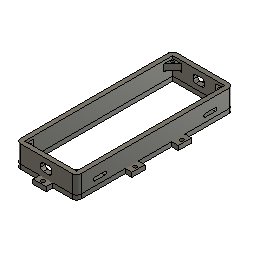
Electronics_Enclosure (Autodesk Fusion 360 design; units mm, degrees)
Autodesk Fusion 360 part; units mm, degrees
sketch "Sketch1" plane through (0, 0, 0) normal (0, 1, 0) x (1, 0, 0)
  line L0 (0, 0) -> (59.69, 0)
  line L1 (59.69, 0) -> (59.69, -170.18)
  line L2 (59.69, -170.18) -> (0, -170.18)
  line L3 (0, -170.18) -> (0, 0)
  line L4 (64.77, 5.08) -> (-5.08, 5.08)
  line L5 (-5.08, 5.08) -> (-5.08, -175.26)
  line L6 (-5.08, -175.26) -> (64.77, -175.26)
  line L7 (64.77, -175.26) -> (64.77, 5.08)
  line L8 (-5.08, -66.04) -> (-5.08, -50.8)
  line L9 (64.77, -85.09) -> (-5.08, -85.09) construction
  line L10 (-5.08, -66.04) -> (-5.08, -50.8)
  line L11 (29.845, -175.26) -> (29.845, 5.08) construction
  line L12 (64.77, -50.8) -> (72.39, -50.8)
  circle A0 centre (68.58, -58.42) radius 2.032
  line L13 (72.39, -50.8) -> (72.39, -66.04)
  line L14 (72.39, -66.04) -> (64.77, -66.04)
  line L15 (64.77, -119.38) -> (72.39, -119.38)
  line L16 (72.39, -119.38) -> (72.39, -104.14)
  line L17 (72.39, -104.14) -> (64.77, -104.14)
  circle A1 centre (68.58, -111.76) radius 2.032
  line L18 (37.465, 5.08) -> (22.225, 5.08)
  line L19 (22.225, 5.08) -> (22.225, 12.7)
  line L20 (22.225, 12.7) -> (37.465, 12.7)
  line L21 (37.465, 12.7) -> (37.465, 5.08)
  line L22 (29.845, 5.08) -> (29.845, 12.7) construction
  circle A2 centre (29.845, 8.89) radius 2.032
  line L23 (22.225, -175.26) -> (22.225, -182.88)
  line L24 (22.225, -182.88) -> (37.465, -182.88)
  line L25 (37.465, -182.88) -> (37.465, -175.26)
  circle A3 centre (29.845, -179.07) radius 2.032
  dimension "d1" = 170.18
  dimension "d2" = 59.69
  dimension "d3" = 5.08
  dimension "d4" = 5.08
  dimension "d5" = 5.08
  dimension "d6" = 5.08
  dimension "d11" = 15.24
  dimension "d12" = 7.62
  dimension "d13" = 4.064
  dimension "d44" = 15.24
  dimension "d45" = 7.62
  dimension "d46" = 7.62
  dimension "d47" = 15.24
  dimension "d48" = 38.1
  dimension "d49" = 55.88
  dimension "d50" = 7.62
  dimension "d51" = 3.81
  dimension "d52" = 4.064
  dimension "d53" = 4.064
  dimension "d54" = 7.62
  dimension "d55" = 3.81
  constraint horizontal L0
  constraint vertical L1
  constraint horizontal L2
  constraint vertical L3
  constraint coincident L0.start L3.end
  constraint horizontal L4
  constraint vertical L5
  constraint horizontal L6
  constraint vertical L7
  constraint vertical L8
  constraint coincident L5 L8.end
  constraint midpoint L7 L9.start
  constraint midpoint L5 L9.end
  constraint midpoint L6 L11.start
  constraint midpoint L4 L11.end
  constraint symmetric L8.end L11 L12.start
  constraint symmetric L8.start L11 L14.end
  constraint horizontal L18
  constraint vertical L19
  constraint horizontal L20
  constraint vertical L21
  constraint coincident L4 L18.start
  constraint midpoint L18 L11.end
  constraint midpoint L20 L22.end
  constraint coincident L11.end L22.start
  constraint midpoint L22 A2.centre
  constraint symmetric L9 L18.start L25.end
  constraint symmetric L9 L18.end L23.start
  constraint symmetric L9 L19.end L23.end
  constraint symmetric L9 L20.end L24.end
  constraint symmetric L9 A2 A3
  constraint perpendicular L7 L14
  constraint perpendicular L13 L14
  constraint perpendicular L7 L15
  constraint perpendicular L15 L16
  constraint coincident L7 L17.end
  measures "d1" distance of L0.start L2.end
  measures "d2" distance of L0.start L0.end
  measures "d3" distance of L1 L7
  measures "d4" distance of L3 L5
  measures "d5" distance of L2 L6
  measures "d6" distance of L0 L4
  measures "d11" distance of L18.start L18.end
  measures "d12" distance of L18.start L20.end
  measures "d13" diameter of A2
  measures "d44" distance of L12.end L13.end
  measures "d45" distance of L12.start L12.end
  measures "d46" distance of L16.end L17.end
  measures "d47" distance of L15.end L16.end
  measures "d48" distance of L14 L17
  measures "d49" distance of L4 L12
  measures "d50" distance of L15 A1.centre
  measures "d51" distance of L16 A1.centre
  measures "d52" diameter of A1
  measures "d53" diameter of A0
  measures "d54" distance of A0.centre L14
  measures "d55" distance of A0.centre L13
extrude "Extrude2" add sketch "Sketch1" along normal blind 5.08 makes body 1
extrude "Extrude1" add sketch "Sketch1" along normal blind 25.4 separate body contours L4 L5 L6 L7 L8 L10 L18 makes body 2
sketch "Sketch2" plane through (0, 25.4, 0) normal (0, 1, 0) x (-1, 0, 0)
  line L0 (-59.69, 170.18) -> (0, 170.18)
  line L1 (0, 170.18) -> (0, 0)
  line L2 (0, 0) -> (-59.69, 0)
  line L3 (-59.69, 0) -> (-59.69, 170.18)
  line L4 (5.08, -5.08) -> (5.08, 175.26)
  line L5 (5.08, 175.26) -> (-64.77, 175.26)
  line L6 (-64.77, 175.26) -> (-64.77, -5.08)
  line L7 (-64.77, -5.08) -> (5.08, -5.08)
ref_plane "WorkPlane1" through (29.845, 22.225, 85.09) normal (0, 1, 0) x (-1, 0, 0)
sketch "Sketch4" plane through (29.845, 22.225, 85.09) normal (0, 1, 0) x (1, 0, 0)
  line L0 (-29.845, 85.09) -> (29.845, 85.09)
  line L1 (29.845, 85.09) -> (29.845, -85.09)
  line L2 (19.685, 85.09) -> (29.845, 74.93)
  line L3 (29.845, 85.09) -> (19.685, 85.09)
  line L4 (29.845, -85.09) -> (19.685, -85.09)
  line L5 (19.685, -85.09) -> (29.845, -74.93)
  line L6 (29.845, -85.09) -> (29.845, -74.93)
  line L7 (-29.845, -85.09) -> (-29.845, 85.09)
  line L8 (-29.845, 85.09) -> (-19.685, 85.09)
  line L9 (-29.845, 85.09) -> (-29.845, 74.93)
  line L10 (-29.845, 74.93) -> (-19.685, 85.09)
  line L11 (29.845, -85.09) -> (-29.845, -85.09)
  line L12 (-29.845, -85.09) -> (-29.845, -74.93)
  line L13 (-29.845, -85.09) -> (-19.685, -85.09)
  line L14 (-19.685, -85.09) -> (-29.845, -74.93)
  circle A0 centre (26.9059, 82.1509) radius 1.651
  line L15 (29.845, 85.09) -> (24.765, 80.01) construction
  line L16 (0, 85.09) -> (0, -85.09) construction
  line L17 (29.845, 0) -> (-29.845, 0) construction
  line L18 (-29.845, 0) -> (29.845, 0) construction
  circle A1 centre (-26.9059, 82.1509) radius 1.651
  circle A2 centre (26.9059, -82.1509) radius 1.651
  circle A3 centre (-26.9059, -82.1509) radius 1.651
  line L19 (29.845, 74.93) -> (29.845, 85.09)
  dimension "d19" = 10.16
  dimension "d20" = 10.16
  dimension "d21" = 10.16
  dimension "d22" = 10.16
  dimension "d23" = 10.16
  dimension "d24" = 10.16
  dimension "d25" = 10.16
  dimension "d26" = 10.16
  dimension "d27" = 3.302
  constraint coincident L0 L2.start
  constraint coincident L1 L2.end
  constraint coincident L0.end L1.start
  constraint coincident L1.end L4.start
  constraint perpendicular L1 L4
  constraint coincident L1 L5.end
  constraint coincident L0.start L7.end
  constraint perpendicular L7 L8
  constraint perpendicular L8 L9
  constraint coincident L7.start L11.end
  constraint perpendicular L11 L12
  constraint perpendicular L7 L13
  constraint midpoint L2 L15.end
  constraint coincident A0.centre L15
  constraint midpoint L0 L16.start
  constraint midpoint L11 L16.end
  constraint midpoint L1 L17.start
  constraint midpoint L7 L17.end
  constraint symmetric A0 L16 A1
  constraint symmetric L16 L17.start L17.end
  constraint symmetric L16 L17.end L17.start
  constraint symmetric A0 L17 A2
  constraint symmetric L17 A1 A3
  measures "d19" distance of L2.start L0.end
  measures "d20" distance of L2.end L3
  measures "d21" distance of L1.end L4.end
  measures "d22" distance of L1.end L5.end
  measures "d23" distance of L0.start L8.end
  measures "d24" distance of L0.start L9.end
  measures "d25" distance of L7.start L12.end
  measures "d26" distance of L7.start L13.end
  measures "d27" diameter of A0
extrude "Extrude3" add sketch "Sketch4" against normal blind 6.35 contours L0 L7 L8 L9 L10 | L0 L1 L2 L3 L19 | L7 L11 L12 L13 L14 | L1 L4 L5 L6 L11 bodies 2
sketch "Sketch7" plane through (0, 0, 175.26) normal (0, 0, 1) x (1, 0, 0)
  line L0 (-5.08, 0) -> (64.77, 0)
  line L1 (64.77, 0) -> (64.77, 25.4)
  line L2 (64.77, 25.4) -> (-5.08, 25.4)
  line L3 (-5.08, 25.4) -> (-5.08, 0)
  line L4 (37.465, 5.08) -> (22.225, 5.08)
  line L5 (29.845, 25.4) -> (29.845, 5.08) construction
  line L6 (36.195, 10.795) -> (23.495, 10.795)
  line L7 (23.495, 10.795) -> (23.495, 19.685)
  line L8 (23.495, 19.685) -> (36.195, 19.685)
  line L9 (36.195, 19.685) -> (36.195, 10.795)
  line L10 (36.195, 10.795) -> (23.495, 19.685) construction
  line L11 (23.495, 10.795) -> (36.195, 19.685) construction
  point P0 (29.845, 15.24)
  dimension "d60" = 12.7
  dimension "d61" = 8.89
  dimension "d66" = 15.24
  constraint midpoint L2 L5.start
  constraint midpoint L4 L5.end
  constraint perpendicular L6 L7
  constraint parallel L6 L8
  constraint parallel L7 L9
  constraint horizontal L6
  constraint coincident L10 P0
  constraint coincident L11 P0
  constraint coincident L5 P0
  measures "d60" distance of L7.end L8.end
  measures "d61" distance of L6.end L7.end
  measures "d66" distance of L0 P0
extrude "Extrude6" cut sketch "Sketch7" against normal blind 230.106 contours L6 L7 L8 L9 bodies 2
fillet "Fillet3" radius 2.921 4 edges at (23.495, 19.685, 172.72) (36.195, 19.685, 172.72) (36.195, 10.795, 172.72) (23.495, 10.795, 172.72) on bodies 2
fillet "Fillet3" radius 2.921 4 edges at (36.195, 19.685, -2.54) (23.495, 19.685, -2.54) (23.495, 10.795, -2.54) (36.195, 10.795, -2.54) on bodies 2
sketch "Sketch6" plane through (64.77, 0, 0) normal (1, 0, 0) x (0, 0, -1)
  line L0 (-175.26, 0) -> (5.08, 0)
  line L1 (5.08, 0) -> (5.08, 25.4)
  line L2 (5.08, 25.4) -> (-175.26, 25.4)
  line L3 (-175.26, 25.4) -> (-175.26, 0)
  line L4 (-140.97, 10.16) -> (-156.21, 10.16)
  line L5 (-156.21, 10.16) -> (-156.21, 13.97)
  line L6 (-156.21, 13.97) -> (-140.97, 13.97)
  line L7 (-140.97, 13.97) -> (-140.97, 10.16)
  line L8 (-85.09, 25.4) -> (-85.09, 0) construction
  line L9 (-29.21, 13.97) -> (-29.21, 10.16)
  line L10 (-13.97, 13.97) -> (-29.21, 13.97)
  line L11 (-29.21, 10.16) -> (-13.97, 10.16)
  line L12 (-13.97, 10.16) -> (-13.97, 13.97)
  dimension "d36" = 15.24
  dimension "d37" = 3.81
  dimension "d38" = 19.05
  dimension "d39" = 11.43
  constraint horizontal L4
  constraint vertical L5
  constraint horizontal L6
  constraint vertical L7
  constraint midpoint L2 L8.start
  constraint midpoint L0 L8.end
  constraint symmetric L4.start L8 L9.end
  constraint symmetric L4.end L8 L11.end
  constraint symmetric L5.end L8 L10.start
  constraint symmetric L6.end L8 L9.start
  measures "d36" distance of L4.start L4.end
  measures "d37" distance of L4.start L6.end
  measures "d38" distance of L3 L5
  measures "d39" distance of L2 L6
extrude "Extrude5" cut sketch "Sketch6" against normal blind 25.5016 contours L4 L5 L6 L7 | L9 L10 L11 L12 bodies 2
fillet "Fillet4" radius 1.778 8 edges at (62.23, 13.97, 140.97) (62.23, 13.97, 156.21) (62.23, 10.16, 156.21) (62.23, 10.16, 140.97) (62.23, 10.16, 13.97) (62.23, 13.97, 13.97) (62.23, 13.97, 29.21) (62.23, 10.16, 29.21) on bodies 2
fillet "Fillet5" radius 5.08 4 edges at (64.77, 12.7, 175.26) (-5.08, 12.7, 175.26) (-5.08, 12.7, -5.08) (64.77, 12.7, -5.08) on bodies 2
fillet "Fillet6" radius 5.08 4 edges at (-5.08, 2.54, -5.08) (64.77, 2.54, -5.08) (64.77, 2.54, 175.26) (-5.08, 2.54, 175.26) on bodies 1
fillet "Fillet2" radius 1.905 8 edges at (59.69, 15.875, 5.08) (54.61, 15.875, 0) (54.61, 15.875, 170.18) (59.69, 15.875, 165.1) (5.08, 15.875, 170.18) (0, 15.875, 165.1) (5.08, 15.875, 0) (0, 15.875, 5.08) on bodies 2
equation "d18 = ( -1 / 8 ) * 1 in"
